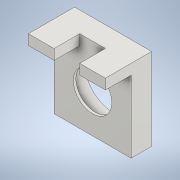
# Autodesk Inventor part: mocowanie lozyska 10-1
Saved by Autodesk Inventor 2021 (Build 250183000, 183)
## iProperties
Created: 2021-11-03
Part Number: mocowanie lozyska 10-1
Material: Generic
Document SubType Name: Modeling
Designer: Łukasz
Density: 1 g/cm^3
Appearance: Steel
Author: Łukasz
Autodesk Inventor part; units mm, degrees
ref_plane "YZ Plane" through (0, 0, 0) normal (1, 0, 0) x (0, 1, 0)
ref_plane "XZ Plane" through (0, 0, 0) normal (0, 1, 0) x (-1, 0, 0)
ref_plane "XY Plane" through (0, 0, 0) normal (0, 0, 1) x (1, 0, 0)
sketch "Sketch1" plane through (0, 0, 0) normal (0, 0, 1) x (1, 0, 0)
  circle A0 centre (0, 0) radius 11.1
  circle A1 centre (0, 0) radius 15
  line L0 (-15, 15) -> (15, 15)
  line L1 (15, 15) -> (15, -15)
  line L2 (15, -15) -> (-15, -15)
  line L3 (-15, -15) -> (-15, 15)
  dimension "d0" = 22.2
  dimension "d1" = 30
  constraints: 8 end point, 2 centre point, 2 coincident, 2 parallel, 1 horizontal, 1 perpendicular
  measures "d0" diameter of A0
  measures "d1" diameter of A1
extrude "Extrusion1" add sketch "Sketch1" along normal blind 7
sketch "Sketch2" plane through (0, 0, 7) normal (0, 0, 1) x (1, 0, 0)
  circle A0 centre (0, 0) radius 7.5
  line L0 (-15, -15) -> (15, -15) projected
  line L1 (15, -15) -> (15, 15) projected
  line L2 (15, 15) -> (-15, 15) projected
  line L3 (-15, 15) -> (-15, -15) projected
  circle A1 centre (0, 0) radius 11.1 projected
  dimension "d4" = 15
  constraints: 1 centre point, 1 coincident
  measures "d4" diameter of A0
extrude "Extrusion2" add sketch "Sketch2" along normal blind 1 contours L3 L2 L1 L0 | A1
sketch "Sketch3" plane through (0, 0, 8) normal (0, 0, 1) x (1, 0, 0)
  line L0 (15, 15) -> (-15, 15) projected
  line L1 (15, -15) -> (15, 15) projected
  line L2 (-15, 15) -> (15, 15)
  line L3 (15, 15) -> (15, 13)
  line L4 (15, 13) -> (-15, 13)
  line L5 (-15, 13) -> (-15, 15)
  point P0 (0, 0)
  dimension "d7" = 2
  constraints: 8 end point, 2 parallel, 1 horizontal, 1 perpendicular, 1 point on line
  measures "d7" distance of L2.end L3.end
extrude "Extrusion3" add sketch "Sketch3" along normal blind 10
sketch "Sketch4" plane through (-15, 15, 0) normal (0, 1, 0) x (1, 0, 0)
  line L0 (0, -18) -> (30, -18) projected
  line L1 (10, -18) -> (20, -18)
  line L2 (20, -18) -> (20, -8)
  line L3 (20, -8) -> (10, -8)
  line L4 (10, -8) -> (10, -18)
  line L5 (0, 0) -> (0, -18) projected
  point P0 (15, 0)
  dimension "d10" = 10
  dimension "d11" = 10
  dimension "d12" = 10
  constraints: 8 end point, 2 parallel, 1 horizontal, 1 perpendicular, 1 point on line
  measures "d10" distance of L3.end L2.end
  measures "d11" distance of L2.end L1.end
  measures "d12" distance between parallel lines of L5 L4
extrude "Extrusion4" cut sketch "Sketch4" against normal blind 10
sketch "Sketch5" plane through (-15, 15, 0) normal (0, 1, 0) x (1, 0, 0)
  line L0 (10, -18) -> (10, -8) projected
  line L1 (10, -8) -> (20, -8) projected
  line L2 (20, -8) -> (20, -18) projected
  line L3 (30, -18) -> (20, -18) projected
  line L4 (30, 0) -> (30, -18) projected
  line L5 (30, 0) -> (0, 0) projected
  line L6 (0, 0) -> (0, -18) projected
  line L7 (10, -18) -> (0, -18) projected
  point P0 (15, 0)
extrude "Extrusion5" add sketch "Sketch5" along normal blind 2
body "Solid1"
